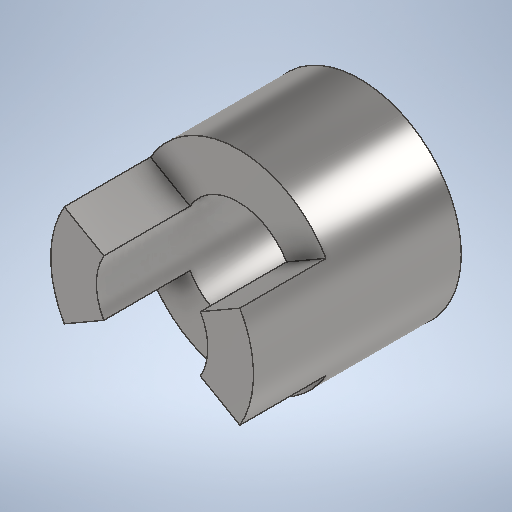
# Autodesk Inventor part: 22MM JAW
Saved by Autodesk Inventor 2025.3 (Build 293356030, 356C)
## iProperties
Created: 2025-10-06
Part Number: 22MM JAW
Material: Generic
Document SubType Name: Modeling
Designer: lstk1ng
Density: 1 g/cm^3
Appearance: Semi-Polished
Author: lstk1ng
Autodesk Inventor part; units mm, degrees
ref_plane "YZ Plane" through (0, 0, 0) normal (1, 0, 0) x (0, 1, 0)
ref_plane "XZ Plane" through (0, 0, 0) normal (0, 1, 0) x (-1, 0, 0)
ref_plane "XY Plane" through (0, 0, 0) normal (0, 0, 1) x (1, 0, 0)
sketch "Sketch1" plane through (0, 0, 0) normal (0, 0, 1) x (1, 0, 0)
  circle A0 centre (0, 0) radius 20
  dimension "d0" = 40
  constraints: 1 centre point, 1 coincident
  measures "d0" diameter of A0
extrude "Extrusion1" add sketch "Sketch1" along normal blind 24
sketch "Sketch2" plane through (0, 0, 24) normal (0, 0, 1) x (1, 0, 0)
  arc A0 (-9.5263, 5.5) -> (-9.5263, -5.5) centre (0, 0) ccw
  line L0 (-9.5263, 5.5) -> (-17.3205, 10)
  circle A1 centre (0, 0) radius 20 projected
  line L1 (0, 0) -> (20, 0) construction
  line L2 (-9.5263, -5.5) -> (-17.3205, -10)
  line L3 (0, 0) -> (20, 0) construction
  line L4 (0, 0) -> (0, 20) construction
  arc A2 (9.5263, -5.5) -> (9.5263, 5.5) centre (0, 0) ccw
  line L5 (9.5263, 5.5) -> (17.3205, 10)
  line L6 (9.5263, -5.5) -> (17.3205, -10)
  dimension "d3" = 22
  dimension "d4" = 150
  dimension "d5" = 150
  constraints: 14 end point, 7 point on circle, 4 symmetric about line, 2 centre point, 2 horizontal, 1 coincident, 1 vertical, 1 other
  measures "d3" diameter of A0
  measures "d4" angle of L1 L0
  measures "d5" angle of L2 L3
extrude "Extrusion2" add sketch "Sketch2" along normal blind 17 contours A0 L2 A1 L0 | A1 L6 A2 L5
sketch "Sketch3" plane through (0, 0, 24) normal (0, 0, 1) x (1, 0, 0)
  circle A0 centre (0, 0) radius 11
  dimension "d8" = 22
  constraints: 1 centre point, 1 coincident
  measures "d8" diameter of A0
extrude "Extrusion3" cut sketch "Sketch3" against normal through all
body "Solid1"
